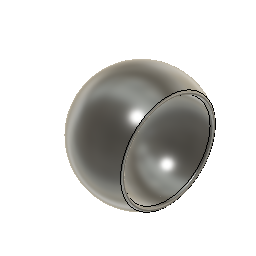
spherica (Autodesk Fusion 360 design; units mm, degrees)
Autodesk Fusion 360 part; units mm, degrees
sphere "SpherePrimitive1" add diameter 125 placed x (1, 0, 0) y (0, 0, -1) z (0, 1, 0) at (0, 0, 0)
sphere "SpherePrimitive2" cut diameter 100 placed x (1, 0, 0) y (0, 1, 0) z (0, 0, 1) at (25, 0, 0)
fillet "Fillet1" radius 2.5 1 edges at (40.625, 17.1752, 44.2817)
sketch "Sketch3" plane through (0, 0, 0) normal (1, 0, 0) x (0, 1, 0)
